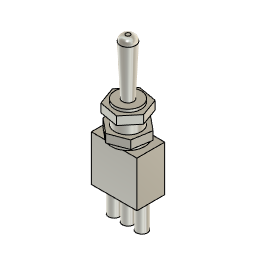
Schalter v5 (Autodesk Fusion 360 design; units mm, degrees)
Autodesk Fusion 360 part; units mm, degrees
sketch "Skizze1" plane through (0, 0, 0) normal (0, 0, 1) x (1, 0, 0)
  line L0 (0, 0) -> (8.2, 0)
  line L1 (8.2, 0) -> (8.2, 5)
  line L2 (8.2, 5) -> (0, 5)
  line L3 (0, 5) -> (0, 0)
  dimension "d1" = 8.2
  dimension "d2" = 5
  constraint horizontal L0
  constraint vertical L1
  constraint horizontal L2
  constraint vertical L3
  constraint coincident L0.start L3.end
  measures "d1" distance of L0.start L0.end
  measures "d2" distance of L0.start L2.end
extrude "Extrusion1" add sketch "Skizze1" along normal blind 8.2
sketch "Skizze2" plane through (0, 0, 8.2) normal (0, 0, 1) x (-1, 0, 0)
  line L0 (0, -5) -> (0, 0)
  line L1 (0, 0) -> (-8.2, 0)
  line L2 (-8.2, 0) -> (-8.2, -5)
  line L3 (-8.2, -5) -> (0, -5)
  circle A0 centre (-4.1, -2.5) radius 3
  dimension "d5" = 6
  dimension "d6" = 2.5
  dimension "d38" = 4.1
  measures "d5" diameter of A0
  measures "d6" distance of L1 A0.centre
  measures "d38" distance of L0 A0.centre
extrude "Extrusion2" add sketch "Skizze2" along normal blind 0.5 contours L3 A0 | L1 L3 A0 | L1 A0
sketch "Skizze3" plane through (0, 0, 8.7) normal (0, 0, 1) x (-1, 0, 0)
  circle A0 centre (-4.1, -2.5) radius 3
  circle A1 centre (-4.1, -2.5) radius 2.375
  dimension "d9" = 4.75
  constraint concentric A0 A1
  measures "d9" diameter of A1
extrude "Extrusion3" add sketch "Skizze3" along normal blind 5.5 contours A1
sketch "Skizze4" plane through (0, 0, 14.2) normal (0, 0, 1) x (-1, 0, 0)
  circle A0 centre (-4.1, -2.5) radius 2.375
  circle A1 centre (-4.1, -2.5) radius 1.25
  dimension "d12" = 2.5
  constraint concentric A0 A1
  measures "d12" diameter of A1
sketch "Skizze5" plane through (0, 0, 0) normal (0, 0, -1) x (1, 0, 0)
  line L0 (0, 0) -> (0, -5)
  line L1 (0, -5) -> (8.2, -5)
  line L2 (8.2, -5) -> (8.2, 0)
  line L3 (8.2, 0) -> (0, 0)
  circle A0 centre (4.1, -2.5) radius 1
  circle A1 centre (6.6, -2.5) radius 1
  circle A2 centre (1.6, -2.5) radius 1
  dimension "d17" = 2
  dimension "d18" = 2.5
  dimension "d21" = 2.5
  dimension "d22" = 0
  dimension "d25" = -2.5
  dimension "d26" = 0
  dimension "d39" = 4.1
  measures "d17" diameter of A0
  measures "d18" distance of L1 A0.centre
  measures "d39" distance of L0 A0.centre
extrude "Extrusion5" add sketch "Skizze5" along normal blind 5 contours A0 | A1 | A2
sketch "Skizze6" plane through (0, 0, 8.7) normal (0, 0, 1) x (-1, 0, 0)
  circle A0 centre (-4.1, -2.5) radius 2.375
  circle A1 centre (-4.1, -2.5) radius 3
  line L0 (-7.3757, -3.7328) -> (-4.6702, -5.9532)
  line L1 (-4.6702, -5.9532) -> (-1.3945, -4.7204)
  line L2 (-1.3945, -4.7204) -> (-0.8243, -1.2672)
  line L3 (-0.8243, -1.2672) -> (-3.5298, 0.9532)
  line L4 (-3.5298, 0.9532) -> (-6.8055, -0.2796)
  line L5 (-6.8055, -0.2796) -> (-7.3757, -3.7328)
  point P0 (-4.1, -2.5)
  dimension "d29" = 3.5
  constraint coincident P0 A0.centre
  measures "d29" distance of L0.start P0
extrude "Extrusion6" add sketch "Skizze6" along normal blind 1.5 contours A1 | L0 L1 L2 L3 L4 L5
ref_plane "Arbeitsebene1" through (4.1, 2.5, 12.2) normal (0, 0, 1) x (-1, 0, 0)
sketch "Skizze8" plane through (4.1, 2.5, 12.2) normal (0, 0, 1) x (1, 0, 0)
  line L0 (-1.1793, 3.2572) -> (-3.4105, 0.6073)
  line L1 (-3.4105, 0.6073) -> (-2.2311, -2.6499)
  line L2 (-2.2311, -2.6499) -> (1.1793, -3.2572)
  line L3 (1.1793, -3.2572) -> (3.4105, -0.6073)
  line L4 (3.4105, -0.6073) -> (2.2311, 2.6499)
  line L5 (2.2311, 2.6499) -> (-1.1793, 3.2572)
  dimension "d40" = 3
  measures "d40" distance of origin L5
extrude "Extrusion9" add sketch "Skizze8" along normal blind 1.5
sketch "Skizze9" plane through (0, 0, 14.2) normal (0, 0, 1) x (-1, 0, 0)
  circle A0 centre (-4.1, -2.5) radius 2.375
  circle A1 centre (-4.1, -2.5) radius 1
  dimension "d43" = 2
  constraint concentric A0 A1
  measures "d43" diameter of A1
extrude "Extrusion10" add sketch "Skizze9" along normal blind 10 draft 2.5 contours A1
fillet "Abrundung2" radius 1 1 edges at (5.4394, 1.9805, 24.2)
